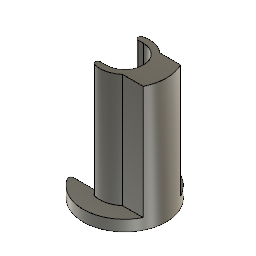
bearing_12mm_extractor v4 (Autodesk Fusion 360 design; units mm, degrees)
Autodesk Fusion 360 part; units mm, degrees
sketch "Sketch1" plane through (0, 0, 0) normal (0, 0, 1) x (1, 0, 0)
  circle A0 centre (0, 0) radius 6.75
  circle A1 centre (0, 0) radius 9
  line L0 (0, -9) -> (0, 9) construction
  circle A2 centre (0, 0) radius 15
  line L1 (0, 6.75) -> (-13.3954, 6.75)
  line L2 (0, -6.75) -> (-13.3954, -6.75)
  line L3 (0, 6.75) -> (13.3954, 6.75)
  line L4 (0, -6.75) -> (13.3954, -6.75)
  dimension "d1" = 13.5
  dimension "d2" = 18
  dimension "d7" = 30
  constraint coincident A0.centre A1.centre
  constraint concentric A0 A1
  constraint coincident A1 L0.start
  constraint coincident A1 L0.end
  constraint vertical L0
  constraint coincident A0 L1.start
  constraint coincident L0 L1.start
  constraint coincident A2 L1.end
  constraint tangent A0 L1
  constraint perpendicular L0 L1
  constraint coincident A0 L2.start
  constraint coincident L0 L2.start
  constraint coincident A2 L2.end
  constraint tangent A0 L2
  constraint coincident A2 L3.end
  constraint tangent A0 L3
  constraint coincident A2 L4.end
  constraint tangent A0 L4
  measures "d1" diameter of A0
  measures "d2" diameter of A1
  measures "d7" diameter of A2
extrude "Extrude4" add sketch "Sketch1" along normal blind 45 contours A0 A1 L3 L4 | A1 L1 L3 | A1 L2 L4 | A1 A2 L3 L4
extrude "Extrude3" add sketch "Sketch1" along normal blind 4 contours A0 A1 L3 L4 | A1 L1 L3 | A1 L2 L4 | A1 A2 L1 L3 | A1 A2 L3 L4 | A1 A2 L2 L4
fillet "Fillet1" radius 1 4 edges at (-5.9529, 6.75, 24.5) (-5.9529, -6.75, 24.5) (-13.3954, 6.75, 2) (-13.3954, -6.75, 2)
